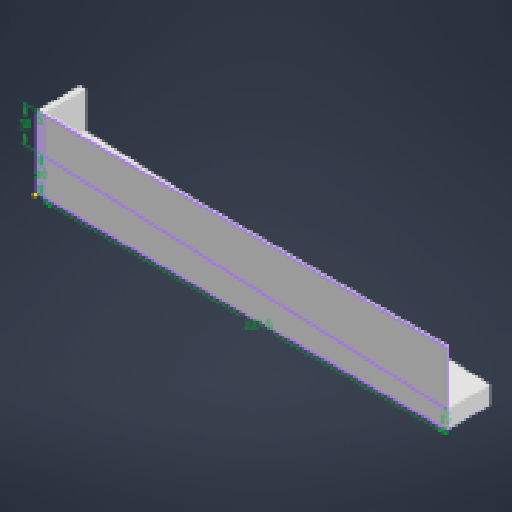
# Autodesk Inventor part: collectingslide
Saved by Autodesk Inventor 2026.2 (Build 302298000, 298)
## iProperties
Created: 2026-03-08
Part Number: collectingslide
Material: Generic
Document SubType Name: Modeling
Designer: danda
Density: 1 g/cm^3
Appearance: Default
Author: danda
Autodesk Inventor part; units mm, degrees
ref_plane "YZ Plane" through (0, 0, 0) normal (1, 0, 0) x (0, 1, 0)
ref_plane "XZ Plane" through (0, 0, 0) normal (0, 1, 0) x (-1, 0, 0)
ref_plane "XY Plane" through (0, 0, 0) normal (0, 0, 1) x (1, 0, 0)
sketch "Sketch1" plane through (0, 0, 0) normal (0, 0, 1) x (1, 0, 0)
  line L0 (6.4984, 1.7965) -> (6.4984, 46.7965)
  line L1 (6.4984, 1.7965) -> (343.9984, 1.7965)
  line L2 (343.9984, 1.7965) -> (343.9984, 36.7965)
  line L3 (343.9984, 36.7965) -> (6.4984, 46.7965)
  line L4 (6.4984, 46.7965) -> (6.4984, 76.7965)
  line L5 (6.4984, 76.7965) -> (343.9984, 76.7965)
  line L6 (343.9984, 76.7965) -> (343.9984, 36.7965)
  line L7 (6.4984, 76.7965) -> (1.4984, 76.7965)
  line L8 (1.4984, 76.7965) -> (1.4984, 1.7965)
  line L9 (1.4984, 1.7965) -> (6.4984, 1.7965)
  point P0 (0, 0)
  dimension "d0" = 45
  dimension "d1" = 35
  dimension "d2" = 337.5
  dimension "d3" = 30
  dimension "d12" = 5
  constraints: 20 end point, 4 perpendicular, 3 vertical, 2 horizontal
  measures "d0" distance of L0.start L0.end
  measures "d1" distance of L1.end L2.end
  measures "d2" distance of L0.start L1.end
  measures "d3" distance of L0.end L4.end
  measures "d12" distance of L4.end L7.end
extrude "Extrusion1" add sketch "Sketch1" against normal blind 45 contours L0 L3 L2 L1
extrude "Extrusion3" add sketch "Sketch1" against normal blind 5 contours L4 L5 L6 L3
extrude "Extrusion5" add sketch "Sketch1" against normal blind 45 contours L9 L8 L7 L4 L0
body "Solid1"
